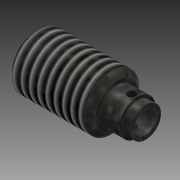
# Autodesk Inventor part: worm_1_20_conrad_with_bolt_hole
Saved by Autodesk Inventor 2017 SP1 (Build 210196100, 196)
## iProperties
Created: 2017-06-26
Part Number: worm_1_20_conrad_with_bolt_hole
Material: Steel
Document SubType Name: Modeling
Designer: JT
Density: 7.85 g/cm^3
Appearance: Plate
Author: JT
Autodesk Inventor part; units mm, degrees
ref_plane "YZ Plane" through (0, 0, 0) normal (1, 0, 0) x (0, 1, 0)
ref_plane "XZ Plane" through (0, 0, 0) normal (0, 1, 0) x (-1, 0, 0)
sketch "Sketch1" plane through (0, 0, 0) normal (0, 0, 1) x (1, 0, 0)
  line L0 (0, 0) -> (0, 4.975)
  line L1 (0, 4.975) -> (15, 4.975)
  line L2 (15, 4.975) -> (15, 3.25)
  line L3 (15, 3.25) -> (20.2, 3.25)
  line L4 (20.2, 3.25) -> (20.2, 0)
  line L5 (20.2, 0) -> (0, 0)
  dimension "d2" = 20.2
  dimension "d3" = 15
  dimension "d19" = 9.95
  dimension "d20" = 6.5
  constraints: 12 end point, 5 perpendicular, 1 vertical
  measures "d2" distance of L4.end L0.start
  measures "d3" distance of L0.end L1.end
  measures "d19" diameter of L1 L5
  measures "d20" diameter of L3 L5
revolve "Revolution1" add sketch "Sketch1" angle 360 about axis through (20.2, 0, 0) along (-1, 0, 0)
thread "Thread1" size "M10x1.5" class "6g" standard "ANSI Metric M Profile" full length
chamfer "Chamfer1" distance 1 angle 45 2 edges at (15, -4.975, 0) (0, -4.975, 0)
hole "Hole1" at (20.2, 0, 0) direction (-1, 0, 0) diameter 4 end through all
ref_plane "Work Plane1" through (17.6, 0, -3.25) normal (0, 0, 1) x (1, 0, 0)
sketch "Sketch2" plane through (17.6, 0, -3.25) normal (0, 0, 1) x (1, 0, 0)
  line L0 (2.6, -3.25) -> (2.6, 3.25) projected
  line L1 (-2.6, -3.25) -> (-2.6, 3.25) projected
  point P0 (-17.6, 0)
  point P1 (0.1, 0)
  point P2 (2.6, 0)
  dimension "d21" = 2.5
  constraints: 1 horizontal alignment, 1 midpoint
  measures "d21" distance of point (0.1, 0) point (2.6, 0)
hole "Hole2" at (17.7, 0, -3.25) direction (0, 0, 1) diameter 1.5 end through all
sketch "Sketch3" plane through (20.2, 0, 0) normal (1, 0, 0) x (0, 0, -1)
  circle A0 centre (0, 0) radius 2.75
  circle A1 centre (0, 0) radius 3.25 projected
  dimension "d29" = 5.5
  constraints: 1 centre point, 1 coincident
  measures "d29" diameter of A0
extrude "Extrusion1" cut sketch "Sketch3" against normal blind 1.5
body "Solid1"
